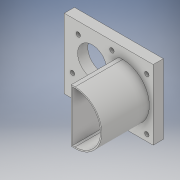
# Autodesk Inventor part: BLOQUE_PARA_MOTOR
Saved by Autodesk Inventor 2019 (Build 230136000, 136)
## iProperties
Created: 2020-09-10
Part Number: BLOQUE_PARA_MOTOR
Material: Generic
Document SubType Name: Modeling
Designer: ASUS
Density: 1 g/cm^3
Appearance: Default
Author: ASUS
Autodesk Inventor part; units mm, degrees
ref_plane "YZ Plane" through (0, 0, 0) normal (1, 0, 0) x (0, 1, 0)
ref_plane "XZ Plane" through (0, 0, 0) normal (0, 1, 0) x (-1, 0, 0)
ref_plane "XY Plane" through (0, 0, 0) normal (0, 0, 1) x (1, 0, 0)
sketch "Sketch1" plane through (0, 0, 0) normal (0, 0, 1) x (1, 0, 0)
  line L0 (0, 0) -> (70, 0)
  line L1 (70, 0) -> (70, 55)
  line L2 (70, 55) -> (0, 55)
  line L3 (0, 55) -> (0, 0)
  dimension "d0" = 70
  dimension "d1" = 55
  constraints: 8 end point, 2 parallel, 1 horizontal, 1 perpendicular
  measures "d0" distance of L2.end L1.end
  measures "d1" distance of L1.end L0.end
extrude "Extrusion1" add sketch "Sketch1" along normal blind 8
sketch "Sketch2" plane through (0, 0, 8) normal (0, 0, 1) x (1, 0, 0)
  circle A0 centre (11, 5) radius 1.75
  circle A1 centre (65, 5) radius 1.75
  circle A2 centre (11, 46) radius 1.75
  circle A3 centre (65, 46) radius 1.75
  line L0 (0, 55) -> (0, 0) projected
  line L1 (0, 0) -> (70, 0) projected
  line L2 (70, 55) -> (0, 55) projected
  line L3 (70, 0) -> (70, 55) projected
  dimension "d4" = 3.5
  dimension "d5" = 3.5
  dimension "d6" = 3.5
  dimension "d7" = 3.5
  dimension "d8" = 11
  dimension "d9" = 5
  dimension "d10" = 9
  dimension "d11" = 5
  constraints: 4 centre point, 2 horizontal alignment, 2 vertical alignment
  measures "d4" diameter of A0
  measures "d5" diameter of A2
  measures "d6" diameter of A3
  measures "d7" diameter of A1
  measures "d8" distance from line of L0 A0.centre
  measures "d9" distance from line of L1 A0.centre
  measures "d10" distance from line of L2 A2.centre
  measures "d11" distance from line of L3 A3.centre
extrude "Extrusion2" cut sketch "Sketch2" against normal blind 40 contours A0 | A1 | A2 | A3
sketch "Sketch3" plane through (0, 0, 0) normal (0, 0, -1) x (-1, 0, 0)
  circle A0 centre (-22, 33) radius 11.5
  line L0 (0, 55) -> (0, 0) projected
  line L1 (-70, 55) -> (0, 55) projected
  dimension "d14" = 23
  dimension "d15" = 22
  dimension "d16" = 22
  constraints: 1 centre point
  measures "d14" diameter of A0
  measures "d15" distance from line of L0 A0.centre
  measures "d16" distance from line of L1 A0.centre
extrude "Extrusion3" cut sketch "Sketch3" against normal blind 35
sketch "Sketch4" plane through (0, 0, 0) normal (0, 0, -1) x (-1, 0, 0)
  circle A0 centre (-22, 33) radius 11.5 projected
  point P0 (0, 0)
  point P1 (-6.5, 48.5)
  point P2 (-37.5, 48.5)
  point P3 (-37.5, 17.5)
  point P4 (-6.5, 17.5)
  dimension "d19" = 15.5
  dimension "d20" = 15.5
  dimension "d21" = 15.5
  dimension "d22" = 15.5
  constraints: 2 horizontal alignment, 2 vertical alignment
  measures "d19" horizontal distance of A0.centre point (-6.5, 48.5)
  measures "d20" horizontal distance of point (-37.5, 48.5) A0.centre
  measures "d21" horizontal distance of point (-37.5, 48.5) A0.centre
  measures "d22" horizontal distance of point (-37.5, 17.5) A0.centre
hole "Hole1" at (6.5, 17.5, 0) at (37.5, 17.5, 0) at (37.5, 48.5, 0) direction (0, 0, 1) diameter 3.5 end through all
sketch "Sketch5" plane through (0, 0, 0) normal (0, 0, -1) x (-1, 0, 0)
  arc A0 (-46, 45.5) -> (-46, 5.5) centre (-46, 25.5) ccw
  line L0 (-46, 45.5) -> (-44, 45.5)
  line L1 (-44, 45.5) -> (-44, 5.5)
  line L2 (-44, 5.5) -> (-46, 5.5)
  line L3 (-70, 0) -> (-70, 55) projected
  point P0 (0, 0)
  dimension "d30" = 40
  dimension "d32" = 25.5
  dimension "d33" = 24
  dimension "d34" = 26
  constraints: 6 end point, 2 perpendicular, 2 point on circle, 2 tangent, 1 centre point, 1 horizontal
  measures "d30" distance of L0.end L1.end
  measures "d32" vertical distance of point (0, 0) A0.centre
  measures "d33" distance from line of A0.centre L3
  measures "d34" distance between parallel lines of L3 L1
extrude "Extrusion4" cut sketch "Sketch5" against normal blind 35
sketch "Sketch6" plane through (0, 0, 8) normal (0, 0, 1) x (1, 0, 0)
  arc A0 (46, 5.5) -> (46, 45.5) centre (46, 25.5) ccw projected
  line L0 (46, 5.5) -> (44, 5.5) projected
  line L1 (44, 5.5) -> (44, 45.5) projected
  line L2 (44, 45.5) -> (46, 45.5) projected
  arc A1 (46, 4.5) -> (46, 46.5) centre (46, 25.5) ccw
  line L3 (46, 4.5) -> (43, 4.5)
  line L4 (43, 4.5) -> (43, 46.5)
  line L5 (43, 46.5) -> (46, 46.5)
  line L6 (70, 0) -> (70, 55) projected
  point P0 (0, 0)
  dimension "d37" = 42
  dimension "d38" = 27
  constraints: 6 end point, 2 coincident, 2 horizontal, 2 point on circle, 2 tangent, 1 centre point, 1 perpendicular
  measures "d37" distance of L3.end L4.end
  measures "d38" distance between parallel lines of L6 L4
extrude "Extrusion5" add sketch "Sketch6" along normal blind 37.5
equation "\"d5\" = d4"
equation "\"d6\" = d4"
equation "\"d7\" = d4"
equation "\"d20\" = d19"
equation "\"d21\" = d19"
equation "\"d22\" = d19"
body "Solid1"
